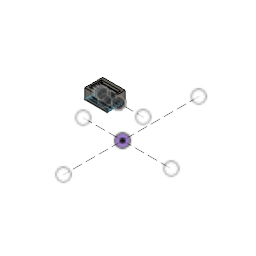
test_print (Autodesk Fusion 360 design; units mm, degrees)
Autodesk Fusion 360 part; units mm, degrees
note: some values were not read from the file. Set by a fixed rule: which sketch regions a step uses.
sketch "Skizze1" plane through (0, 0, 0) normal (0, 0, 1) x (1, 0, 0)
  line L0 (-31.0471, 0) -> (38.3523, 0) construction
  line L1 (0, 60) -> (0, -46.5706) construction
  line L2 (-43.2224, 24.13) -> (-7.914, 24.13) construction
  line L3 (-37.9766, 22.86) -> (-40.5166, 22.86)
  line L4 (-40.5166, 22.86) -> (-40.5166, 25.4)
  line L5 (-40.5166, 25.4) -> (-37.9766, 25.4)
  line L6 (-37.9766, 25.4) -> (-37.9766, 22.86)
  line L7 (-37.9766, 22.86) -> (-40.5166, 25.4) construction
  line L8 (-40.5166, 22.86) -> (-37.9766, 25.4) construction
  line L9 (-38.6466, 23.53) -> (-39.8466, 23.53)
  line L10 (-39.8466, 23.53) -> (-39.8466, 24.73)
  line L11 (-39.8466, 24.73) -> (-38.6466, 24.73)
  line L12 (-38.6466, 24.73) -> (-38.6466, 23.53)
  line L13 (-38.6466, 23.53) -> (-39.8466, 24.73) construction
  line L14 (-39.8466, 23.53) -> (-38.6466, 24.73) construction
  line L15 (-37.9766, 22.86) -> (-37.9766, 25.4)
  line L16 (-37.9766, 25.4) -> (-35.4366, 25.4)
  line L17 (-35.4366, 25.4) -> (-35.4366, 22.86)
  line L18 (-35.4366, 22.86) -> (-37.9766, 22.86)
  line L19 (-37.3066, 23.53) -> (-37.3066, 24.73)
  line L20 (-37.3066, 24.73) -> (-36.1066, 24.73)
  line L21 (-36.1066, 23.53) -> (-37.3066, 23.53)
  line L22 (-36.1066, 24.73) -> (-36.1066, 23.53)
  line L23 (-35.4366, 22.86) -> (-35.4366, 25.4)
  line L24 (-35.4366, 25.4) -> (-32.8966, 25.4)
  line L25 (-32.8966, 25.4) -> (-32.8966, 22.86)
  line L26 (-32.8966, 22.86) -> (-35.4366, 22.86)
  line L27 (-34.7666, 23.53) -> (-34.7666, 24.73)
  line L28 (-34.7666, 24.73) -> (-33.5666, 24.73)
  line L29 (-33.5666, 23.53) -> (-34.7666, 23.53)
  line L30 (-33.5666, 24.73) -> (-33.5666, 23.53)
  line L31 (-32.8966, 22.86) -> (-32.8966, 25.4)
  line L32 (-32.8966, 25.4) -> (-30.3566, 25.4)
  line L33 (-30.3566, 25.4) -> (-30.3566, 22.86)
  line L34 (-30.3566, 22.86) -> (-32.8966, 22.86)
  line L35 (-32.2266, 23.53) -> (-32.2266, 24.73)
  line L36 (-32.2266, 24.73) -> (-31.0266, 24.73)
  line L37 (-31.0266, 23.53) -> (-32.2266, 23.53)
  line L38 (-31.0266, 24.73) -> (-31.0266, 23.53)
  line L39 (-30.3566, 22.86) -> (-30.3566, 25.4)
  line L40 (-30.3566, 25.4) -> (-27.8166, 25.4)
  line L41 (-27.8166, 25.4) -> (-27.8166, 22.86)
  line L42 (-27.8166, 22.86) -> (-30.3566, 22.86)
  line L43 (-29.6866, 23.53) -> (-29.6866, 24.73)
  line L44 (-29.6866, 24.73) -> (-28.4866, 24.73)
  line L45 (-28.4866, 23.53) -> (-29.6866, 23.53)
  line L46 (-28.4866, 24.73) -> (-28.4866, 23.53)
  line L47 (-27.8166, 23.13) -> (-40.5166, 23.13)
  line L48 (-40.5166, 23.13) -> (-40.5166, 25.13)
  line L49 (-40.5166, 25.13) -> (-27.8166, 25.13)
  line L50 (-27.8166, 25.13) -> (-27.8166, 23.13)
  line L51 (-27.8166, 23.13) -> (-40.5166, 25.13) construction
  line L52 (-40.5166, 23.13) -> (-27.8166, 25.13) construction
  line L53 (-40.5166, 20.32) -> (-40.5166, 22.86)
  line L54 (-40.5166, 22.86) -> (-37.9766, 22.86)
  line L55 (-37.9766, 22.86) -> (-37.9766, 20.32)
  line L56 (-37.9766, 20.32) -> (-40.5166, 20.32)
  line L57 (-39.8466, 20.99) -> (-39.8466, 22.19)
  line L58 (-39.8466, 22.19) -> (-38.6466, 22.19)
  line L59 (-38.6466, 20.99) -> (-39.8466, 20.99)
  line L60 (-38.6466, 22.19) -> (-38.6466, 20.99)
  line L61 (-37.9766, 20.32) -> (-37.9766, 22.86)
  line L62 (-37.9766, 22.86) -> (-35.4366, 22.86)
  line L63 (-35.4366, 22.86) -> (-35.4366, 20.32)
  line L64 (-35.4366, 20.32) -> (-37.9766, 20.32)
  line L65 (-37.3066, 20.99) -> (-37.3066, 22.19)
  line L66 (-37.3066, 22.19) -> (-36.1066, 22.19)
  line L67 (-36.1066, 20.99) -> (-37.3066, 20.99)
  line L68 (-36.1066, 22.19) -> (-36.1066, 20.99)
  line L69 (-35.4366, 20.32) -> (-35.4366, 22.86)
  line L70 (-35.4366, 22.86) -> (-32.8966, 22.86)
  line L71 (-32.8966, 22.86) -> (-32.8966, 20.32)
  line L72 (-32.8966, 20.32) -> (-35.4366, 20.32)
  line L73 (-34.7666, 20.99) -> (-34.7666, 22.19)
  line L74 (-34.7666, 22.19) -> (-33.5666, 22.19)
  line L75 (-33.5666, 20.99) -> (-34.7666, 20.99)
  line L76 (-33.5666, 22.19) -> (-33.5666, 20.99)
  line L77 (-32.8966, 20.32) -> (-32.8966, 22.86)
  line L78 (-32.8966, 22.86) -> (-30.3566, 22.86)
  line L79 (-30.3566, 22.86) -> (-30.3566, 20.32)
  line L80 (-30.3566, 20.32) -> (-32.8966, 20.32)
  line L81 (-32.2266, 20.99) -> (-32.2266, 22.19)
  line L82 (-32.2266, 22.19) -> (-31.0266, 22.19)
  line L83 (-31.0266, 20.99) -> (-32.2266, 20.99)
  line L84 (-31.0266, 22.19) -> (-31.0266, 20.99)
  line L85 (-30.3566, 20.32) -> (-30.3566, 22.86)
  line L86 (-30.3566, 22.86) -> (-27.8166, 22.86)
  line L87 (-27.8166, 22.86) -> (-27.8166, 20.32)
  line L88 (-27.8166, 20.32) -> (-30.3566, 20.32)
  line L89 (-29.6866, 20.99) -> (-29.6866, 22.19)
  line L90 (-29.6866, 22.19) -> (-28.4866, 22.19)
  line L91 (-28.4866, 20.99) -> (-29.6866, 20.99)
  line L92 (-28.4866, 22.19) -> (-28.4866, 20.99)
  line L93 (-40.5166, 17.78) -> (-40.5166, 20.32)
  line L94 (-40.5166, 20.32) -> (-37.9766, 20.32)
  line L95 (-37.9766, 20.32) -> (-37.9766, 17.78)
  line L96 (-37.9766, 17.78) -> (-40.5166, 17.78)
  line L97 (-39.8466, 18.45) -> (-39.8466, 19.65)
  line L98 (-39.8466, 19.65) -> (-38.6466, 19.65)
  line L99 (-38.6466, 18.45) -> (-39.8466, 18.45)
  line L100 (-38.6466, 19.65) -> (-38.6466, 18.45)
  line L101 (-37.9766, 17.78) -> (-37.9766, 20.32)
  line L102 (-37.9766, 20.32) -> (-35.4366, 20.32)
  line L103 (-35.4366, 20.32) -> (-35.4366, 17.78)
  line L104 (-35.4366, 17.78) -> (-37.9766, 17.78)
  line L105 (-37.3066, 18.45) -> (-37.3066, 19.65)
  line L106 (-37.3066, 19.65) -> (-36.1066, 19.65)
  line L107 (-36.1066, 18.45) -> (-37.3066, 18.45)
  line L108 (-36.1066, 19.65) -> (-36.1066, 18.45)
  line L109 (-35.4366, 17.78) -> (-35.4366, 20.32)
  line L110 (-35.4366, 20.32) -> (-32.8966, 20.32)
  line L111 (-32.8966, 20.32) -> (-32.8966, 17.78)
  line L112 (-32.8966, 17.78) -> (-35.4366, 17.78)
  line L113 (-34.7666, 18.45) -> (-34.7666, 19.65)
  line L114 (-34.7666, 19.65) -> (-33.5666, 19.65)
  line L115 (-33.5666, 18.45) -> (-34.7666, 18.45)
  line L116 (-33.5666, 19.65) -> (-33.5666, 18.45)
  line L117 (-32.8966, 17.78) -> (-32.8966, 20.32)
  line L118 (-32.8966, 20.32) -> (-30.3566, 20.32)
  line L119 (-30.3566, 20.32) -> (-30.3566, 17.78)
  line L120 (-30.3566, 17.78) -> (-32.8966, 17.78)
  line L121 (-32.2266, 18.45) -> (-32.2266, 19.65)
  line L122 (-32.2266, 19.65) -> (-31.0266, 19.65)
  line L123 (-31.0266, 18.45) -> (-32.2266, 18.45)
  line L124 (-31.0266, 19.65) -> (-31.0266, 18.45)
  line L125 (-30.3566, 17.78) -> (-30.3566, 20.32)
  line L126 (-30.3566, 20.32) -> (-27.8166, 20.32)
  line L127 (-27.8166, 20.32) -> (-27.8166, 17.78)
  line L128 (-27.8166, 17.78) -> (-30.3566, 17.78)
  line L129 (-29.6866, 18.45) -> (-29.6866, 19.65)
  line L130 (-29.6866, 19.65) -> (-28.4866, 19.65)
  line L131 (-28.4866, 18.45) -> (-29.6866, 18.45)
  line L132 (-28.4866, 19.65) -> (-28.4866, 18.45)
  line L133 (-40.5166, 15.24) -> (-40.5166, 17.78)
  line L134 (-40.5166, 17.78) -> (-37.9766, 17.78)
  line L135 (-37.9766, 17.78) -> (-37.9766, 15.24)
  line L136 (-37.9766, 15.24) -> (-40.5166, 15.24)
  line L137 (-39.8466, 15.91) -> (-39.8466, 17.11)
  line L138 (-39.8466, 17.11) -> (-38.6466, 17.11)
  line L139 (-38.6466, 15.91) -> (-39.8466, 15.91)
  line L140 (-38.6466, 17.11) -> (-38.6466, 15.91)
  line L141 (-37.9766, 15.24) -> (-37.9766, 17.78)
  line L142 (-37.9766, 17.78) -> (-35.4366, 17.78)
  line L143 (-35.4366, 17.78) -> (-35.4366, 15.24)
  line L144 (-35.4366, 15.24) -> (-37.9766, 15.24)
  line L145 (-37.3066, 15.91) -> (-37.3066, 17.11)
  line L146 (-37.3066, 17.11) -> (-36.1066, 17.11)
  line L147 (-36.1066, 15.91) -> (-37.3066, 15.91)
  line L148 (-36.1066, 17.11) -> (-36.1066, 15.91)
  line L149 (-35.4366, 15.24) -> (-35.4366, 17.78)
  line L150 (-35.4366, 17.78) -> (-32.8966, 17.78)
  line L151 (-32.8966, 17.78) -> (-32.8966, 15.24)
  line L152 (-32.8966, 15.24) -> (-35.4366, 15.24)
  line L153 (-34.7666, 15.91) -> (-34.7666, 17.11)
  line L154 (-34.7666, 17.11) -> (-33.5666, 17.11)
  line L155 (-33.5666, 15.91) -> (-34.7666, 15.91)
  line L156 (-33.5666, 17.11) -> (-33.5666, 15.91)
  line L157 (-32.8966, 15.24) -> (-32.8966, 17.78)
  line L158 (-32.8966, 17.78) -> (-30.3566, 17.78)
  line L159 (-30.3566, 17.78) -> (-30.3566, 15.24)
  line L160 (-30.3566, 15.24) -> (-32.8966, 15.24)
  line L161 (-32.2266, 15.91) -> (-32.2266, 17.11)
  line L162 (-32.2266, 17.11) -> (-31.0266, 17.11)
  line L163 (-31.0266, 15.91) -> (-32.2266, 15.91)
  line L164 (-31.0266, 17.11) -> (-31.0266, 15.91)
  line L165 (-30.3566, 15.24) -> (-30.3566, 17.78)
  line L166 (-30.3566, 17.78) -> (-27.8166, 17.78)
  line L167 (-27.8166, 17.78) -> (-27.8166, 15.24)
  line L168 (-27.8166, 15.24) -> (-30.3566, 15.24)
  line L169 (-29.6866, 15.91) -> (-29.6866, 17.11)
  line L170 (-29.6866, 17.11) -> (-28.4866, 17.11)
  line L171 (-28.4866, 15.91) -> (-29.6866, 15.91)
  line L172 (-28.4866, 17.11) -> (-28.4866, 15.91)
  line L173 (-40.5166, 22.59) -> (-27.8166, 22.59)
  line L174 (-27.8166, 22.59) -> (-27.8166, 20.59)
  line L175 (-27.8166, 20.59) -> (-40.5166, 20.59)
  line L176 (-40.5166, 20.59) -> (-40.5166, 22.59)
  line L177 (-40.5166, 20.05) -> (-27.8166, 20.05)
  line L178 (-27.8166, 20.05) -> (-27.8166, 18.05)
  line L179 (-27.8166, 18.05) -> (-40.5166, 18.05)
  line L180 (-40.5166, 18.05) -> (-40.5166, 20.05)
  line L181 (-40.5166, 17.51) -> (-27.8166, 17.51)
  line L182 (-27.8166, 17.51) -> (-27.8166, 15.51)
  line L183 (-27.8166, 15.51) -> (-40.5166, 15.51)
  line L184 (-40.5166, 15.51) -> (-40.5166, 17.51)
  line L185 (-25.3166, 13.24) -> (-43.0166, 13.24)
  line L186 (-43.0166, 13.24) -> (-43.0166, 27.4)
  line L187 (-43.0166, 27.4) -> (-25.3166, 27.4)
  line L188 (-25.3166, 27.4) -> (-25.3166, 13.24)
  line L189 (-25.3166, 13.24) -> (-43.0166, 27.4) construction
  line L190 (-43.0166, 13.24) -> (-25.3166, 27.4) construction
  line L191 (-27.8166, 23.13) -> (-26.6166, 23.13)
  line L192 (-26.6166, 23.13) -> (-26.6166, 25.13)
  line L193 (-26.6166, 25.13) -> (-27.8166, 25.13)
  line L194 (-27.8166, 25.13) -> (-27.8166, 23.13)
  line L195 (-27.8166, 23.13) -> (-26.6166, 25.13) construction
  line L196 (-26.6166, 23.13) -> (-27.8166, 25.13) construction
  line L197 (-41.7166, 23.13) -> (-40.5166, 23.13)
  line L198 (-40.5166, 23.13) -> (-40.5166, 25.13)
  line L199 (-40.5166, 25.13) -> (-41.7166, 25.13)
  line L200 (-41.7166, 25.13) -> (-41.7166, 23.13)
  line L201 (-41.7166, 23.13) -> (-40.5166, 25.13) construction
  line L202 (-40.5166, 23.13) -> (-41.7166, 25.13) construction
  line L203 (-27.8166, 20.59) -> (-26.6166, 20.59)
  line L204 (-26.6166, 20.59) -> (-26.6166, 22.59)
  line L205 (-27.8166, 22.59) -> (-27.8166, 20.59)
  line L206 (-26.6166, 22.59) -> (-27.8166, 22.59)
  line L207 (-41.7166, 20.59) -> (-40.5166, 20.59)
  line L208 (-40.5166, 20.59) -> (-40.5166, 22.59)
  line L209 (-41.7166, 22.59) -> (-41.7166, 20.59)
  line L210 (-40.5166, 22.59) -> (-41.7166, 22.59)
  line L211 (-27.8166, 18.05) -> (-26.6166, 18.05)
  line L212 (-26.6166, 18.05) -> (-26.6166, 20.05)
  line L213 (-27.8166, 20.05) -> (-27.8166, 18.05)
  line L214 (-26.6166, 20.05) -> (-27.8166, 20.05)
  line L215 (-41.7166, 18.05) -> (-40.5166, 18.05)
  line L216 (-40.5166, 18.05) -> (-40.5166, 20.05)
  line L217 (-41.7166, 20.05) -> (-41.7166, 18.05)
  line L218 (-40.5166, 20.05) -> (-41.7166, 20.05)
  line L219 (-27.8166, 15.51) -> (-26.6166, 15.51)
  line L220 (-26.6166, 15.51) -> (-26.6166, 17.51)
  line L221 (-27.8166, 17.51) -> (-27.8166, 15.51)
  line L222 (-26.6166, 17.51) -> (-27.8166, 17.51)
  line L223 (-41.7166, 15.51) -> (-40.5166, 15.51)
  line L224 (-40.5166, 15.51) -> (-40.5166, 17.51)
  line L225 (-41.7166, 17.51) -> (-41.7166, 15.51)
  line L226 (-40.5166, 17.51) -> (-41.7166, 17.51)
  point P0 (-39.2466, 24.13)
  point P1 (-39.2466, 24.13)
  point P2 (-34.1666, 24.13)
  point P3 (-34.1666, 20.32)
  point P4 (-27.2166, 24.13)
  point P5 (-41.1166, 24.13)
  dimension "d1" = 24.13
  dimension "d2" = 2.54
  dimension "d3" = 2.54
  dimension "d4" = 1.2
  dimension "d5" = 1.2
  dimension "d8" = 10.16
  dimension "d9" = -7.62
  dimension "d11" = 2
  dimension "d12" = 12.7
  dimension "d16" = 0
  dimension "d17" = -7.62
  dimension "d18" = 14.16
  dimension "d19" = 17.7
  dimension "d20" = 2.5
  dimension "d28" = 2
  dimension "d29" = 1.2
  dimension "d30" = 1.2
  dimension "d31" = 2
  constraint horizontal L0
  constraint coincident origin L0
  constraint vertical L1
  constraint coincident origin L1
  constraint parallel L0 L2
  constraint horizontal L3
  constraint perpendicular L3 L4
  constraint parallel L3 L5
  constraint parallel L4 L6
  constraint coincident L7 P1
  constraint coincident L8 P1
  constraint coincident L2 P1
  constraint horizontal L9
  constraint perpendicular L9 L10
  constraint parallel L9 L11
  constraint parallel L10 L12
  constraint coincident L13 P1
  constraint coincident L14 P1
  constraint coincident P1 P0
  constraint horizontal L47
  constraint perpendicular L47 L48
  constraint parallel L47 L49
  constraint parallel L48 L50
  constraint coincident L51 P2
  constraint coincident L52 P2
  constraint coincident L2 P2
  constraint horizontal L185
  constraint perpendicular L185 L186
  constraint parallel L185 L187
  constraint parallel L186 L188
  constraint coincident L189 P3
  constraint coincident L190 P3
  constraint coincident L110 P3
  constraint coincident L41 L49.end
  constraint coincident L4 L48.end
  constraint horizontal L191
  constraint perpendicular L191 L192
  constraint parallel L191 L193
  constraint parallel L192 L194
  constraint coincident L195 P4
  constraint coincident L196 P4
  constraint coincident L2 P4
  constraint horizontal L197
  constraint perpendicular L197 L198
  constraint parallel L197 L199
  constraint parallel L198 L200
  constraint coincident L201 P5
  constraint coincident L202 P5
  constraint coincident L2 P5
  measures "d1" distance of L0 L2
  measures "d2" distance of L4 L6
  measures "d3" distance of L3 L5
  measures "d4" distance of L9 L11
  measures "d5" distance of L10 L12
  measures "d11" distance of L47 L49
  measures "d12" distance of L4 L41
  measures "d18" distance of L185 L187
  measures "d19" distance of L186 L188
  measures "d20" distance of L87 L188
  measures "d28" distance of L191 L193
  measures "d29" distance of L192 L194
  measures "d30" distance of L198 L200
  measures "d31" distance of L197 L199
extrude "Extrusion1" add sketch "Skizze1" along normal blind 1.2 contours L3 L53 L54 L55 L61 L173 | L3 L4 L6 L15 L47 L54 | L6 L15 L17 L18 L23 L47 L62 | L18 L55 L61 L62 L63 L69 L173 | L4 L6 L15 L47 L48 L49 L198 | L6 L15 L17 L23 L47 L49 | L17 L23 L25 L26 L31 L47 L70 | L26 L63 L69 L70 L71 L77 L173 | L55 L61 L63 L69 L173 L175 | L53 L55 L61 L173 L175 L176 L208 | L4 L48 L197 L198 L199 L200 | L53 L176 L207 L208 L209 L210 | L4 L5 L6 L15 L49 | L6 L15 L16 L17 L23 L49 | L17 L23 L25 L31 L47 L49 | L25 L31 L33 L34 L39 L47 L78 | L34 L71 L77 L78 L79 L85 L173 | L63 L69 L71 L77 L173 L175 | L55 L61 L63 L64 L69 L102 L175 | L53 L55 L56 L61 L94 L175 | L17 L23 L24 L25 L31 L49 | L25 L31 L33 L39 L47 L49 | L33 L39 L41 L42 L47 L86 | L42 L79 L85 L86 L87 L173 | L71 L77 L79 L85 L173 L175 | L63 L69 L71 L72 L77 L110 L175 | L56 L93 L94 L95 L101 L177 | L64 L95 L101 L102 L103 L109 L177 | L25 L31 L32 L33 L39 L49 | L33 L39 L41 L47 L49 L50 L194 | L79 L85 L87 L173 L174 L175 L205 | L71 L77 L79 L80 L85 L118 L175 | L72 L103 L109 L110 L111 L117 L177 | L95 L101 L103 L109 L177 L179 | L93 L95 L101 L177 L179 L180 L216 | L93 L180 L215 L216 L217 L218 | L33 L39 L40 L41 L49 | L41 L50 L191 L192 L193 L194 | L87 L174 L203 L204 L205 L206 | L79 L85 L87 L88 L126 L175 | L80 L111 L117 L118 L119 L125 L177 | L103 L109 L111 L117 L177 L179 | L95 L101 L103 L104 L109 L142 L179 | L93 L95 L96 L101 L134 L179 | L88 L119 L125 L126 L127 L177 | L111 L117 L119 L125 L177 L179 | L103 L109 L111 L112 L117 L150 L179 | L96 L133 L134 L135 L141 L181 | L104 L135 L141 L142 L143 L149 L181 | L119 L125 L127 L177 L178 L179 L213 | L111 L117 L119 L120 L125 L158 L179 | L112 L143 L149 L150 L151 L157 L181 | L135 L141 L143 L149 L181 L183 | L133 L135 L141 L181 L183 L184 L224 | L133 L184 L223 L224 L225 L226 | L127 L178 L211 L212 L213 L214 | L119 L125 L127 L128 L166 L179 | L120 L151 L157 L158 L159 L165 L181 | L143 L149 L151 L157 L181 L183 | L135 L141 L143 L144 L149 L183 | L133 L135 L136 L141 L183 | L128 L159 L165 L166 L167 L181 | L151 L157 L159 L165 L181 L183 | L143 L149 L151 L152 L157 L183 | L159 L165 L167 L181 L182 L183 L221 | L151 L157 L159 L160 L165 L183 | L167 L182 L219 L220 L221 L222 | L159 L165 L167 L168 L183 | L185 L186 L187 L188
extrude "Extrusion2" add sketch "Skizze1" along normal blind 8 contours L3 L53 L54 L55 L61 L173 | L3 L4 L6 L15 L47 L54 | L6 L15 L17 L18 L23 L47 L62 | L18 L55 L61 L62 L63 L69 L173 | L17 L23 L25 L26 L31 L47 L70 | L26 L63 L69 L70 L71 L77 L173 | L4 L5 L6 L15 L49 | L6 L15 L16 L17 L23 L49 | L25 L31 L33 L34 L39 L47 L78 | L34 L71 L77 L78 L79 L85 L173 | L55 L61 L63 L64 L69 L102 L175 | L53 L55 L56 L61 L94 L175 | L17 L23 L24 L25 L31 L49 | L33 L39 L41 L42 L47 L86 | L42 L79 L85 L86 L87 L173 | L63 L69 L71 L72 L77 L110 L175 | L56 L93 L94 L95 L101 L177 | L64 L95 L101 L102 L103 L109 L177 | L25 L31 L32 L33 L39 L49 | L71 L77 L79 L80 L85 L118 L175 | L72 L103 L109 L110 L111 L117 L177 | L33 L39 L40 L41 L49 | L79 L85 L87 L88 L126 L175 | L80 L111 L117 L118 L119 L125 L177 | L95 L101 L103 L104 L109 L142 L179 | L93 L95 L96 L101 L134 L179 | L88 L119 L125 L126 L127 L177 | L103 L109 L111 L112 L117 L150 L179 | L96 L133 L134 L135 L141 L181 | L104 L135 L141 L142 L143 L149 L181 | L111 L117 L119 L120 L125 L158 L179 | L112 L143 L149 L150 L151 L157 L181 | L119 L125 L127 L128 L166 L179 | L120 L151 L157 L158 L159 L165 L181 | L135 L141 L143 L144 L149 L183 | L133 L135 L136 L141 L183 | L128 L159 L165 L166 L167 L181 | L143 L149 L151 L152 L157 L183 | L151 L157 L159 L160 L165 L183 | L159 L165 L167 L168 L183 | L185 L186 L187 L188
extrude "Extrusion3" add sketch "Skizze1" along normal blind 6.8 contours L4 L48 L197 L198 L199 L200 | L53 L176 L207 L208 L209 L210 | L93 L180 L215 L216 L217 L218 | L41 L50 L191 L192 L193 L194 | L87 L174 L203 L204 L205 L206 | L133 L184 L223 L224 L225 L226 | L127 L178 L211 L212 L213 L214 | L167 L182 L219 L220 L221 L222
chamfer "Fase3" [suppressed]
equation "d1 = ( 9 * 2.54 ) * 1 mm + 1.27 mm"
equation "d8 = ( 4 * 2.54 ) * 1 mm"
equation "d9 = -3 * 2.540 mm"
equation "d17 = -3 * 2.54000 mm"
equation "d18 = ( 4 * 2.54 ) * 1 mm + 4 mm"
equation "d19 = ( 5 * 2.54 ) * 1 mm + 5 mm"
named bodies: "test1"
